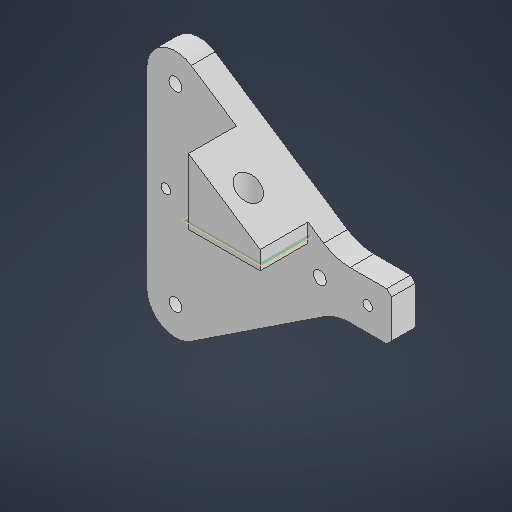
# Autodesk Inventor part: y axis something back
Saved by Autodesk Inventor 2025.1 (Build 291241000, 241)
## iProperties
Created: 2025-02-02
Part Number: y axis something back
Material: Generic
Document SubType Name: Modeling
Designer: jerem
Density: 1 g/cm^3
Appearance: Default
Author: jerem
## iProperties of the stored document y axis something back_3DPrint.ipt
Created: 2025-02-19
Part Number: y axis something back_3DPrint
Material: Generic
Document SubType Name: Modeling
Designer: jerem
Density: 1 g/cm^3
Appearance: Default
Author: jerem
Autodesk Inventor part; units mm, degrees
ref_plane "YZ Plane" through (0, 0, 0) normal (1, 0, 0) x (0, 1, 0)
ref_plane "XZ Plane" through (0, 0, 0) normal (0, 1, 0) x (-1, 0, 0)
ref_plane "XY Plane" through (0, 0, 0) normal (0, 0, 1) x (1, 0, 0)
sketch "Sketch1" plane through (0, 0, 0) normal (0, 0, 1) x (1, 0, 0)
  line L0 (0, 0) -> (30.25, 0) construction
  line L1 (0, 0) -> (-30.25, 0) construction
  line L2 (-30.25, 0) -> (-30.25, 40) construction
  line L3 (-30.25, 0) -> (-30.25, -40) construction
  circle A0 centre (-30.25, 40) radius 2.7
  circle A1 centre (-30.25, -40) radius 2.7
  circle A2 centre (30.25, 0) radius 2.7
  circle A3 centre (-30.25, 40) radius 12
  circle A4 centre (-30.25, -40) radius 12
  circle A5 centre (30.25, 0) radius 12
  line L4 (36.868172, -10.009985) -> (-23.631828, -50.009985)
  line L5 (-42.25, 40) -> (-42.25, -40)
  circle A6 centre (-34.25, 0) radius 2
  line L6 (-30.25, 0) -> (-34.25, 0) construction
  line L7 (-23.631828, 50.009985) -> (36.868172, 10.009985)
  line L8 (30.25, 0) -> (50.25, 0) construction
  circle A7 centre (50.25, 0) radius 10
  circle A8 centre (50.25, 0) radius 2
  line L9 (50.25746, 9.999997) -> (36.868172, 10.009985)
  line L10 (50.25746, -9.999997) -> (36.868172, -10.009985)
  circle A9 centre (10.25, 0) radius 2
  line L11 (50.25746, -9.999997) -> (60.257457, -9.992538)
  line L12 (60.257457, -9.992538) -> (60.242549, 9.992549)
  line L13 (60.242549, 9.992549) -> (50.25746, 9.999997)
  point P0 (-42.25, 0)
  point P1 (41.35, -4.559605)
  point P2 (41.35, 4.559605)
  point P3 (60.249997, 0.00746)
  dimension "d0" = 60.5
  dimension "d1" = 5.4
  dimension "d2" = 80
  dimension "d3" = 24
  dimension "d55" = 4
  dimension "d56" = 8
  dimension "d57" = 20
  dimension "d58" = 20
  dimension "d69" = 20
  constraints: 28 end point, 10 centre point, 10 tangent, 8 coincident, 8 point on circle, 6 equal radius, 4 horizontal, 2 collinear, 2 perpendicular, 2 vertical, 1 midpoint, 1 point on line
  measures "d0" distance of L0.end L1.end
  measures "d1" diameter of A0
  measures "d2" distance of L3.end L2.end
  measures "d3" diameter of A3
  measures "d55" diameter of A6
  measures "d56" distance of point (-42.25, 0) L6.end
  measures "d57" distance of L8.start L8.end
  measures "d58" diameter of A7
  measures "d69" distance of A9.centre L0.end
sketch "Sketch1 outline for Extrusion1" plane through (0, 0, 0) normal (0, 0, 1) x (1, 0, 0)
  arc A0 (-23.631828, 50.009985) -> (-42.25, 40) centre (-30.25, 40) ccw
  line L0 (-42.25, 40) -> (-42.25, -40)
  arc A1 (-42.25, -40) -> (-23.631828, -50.009985) centre (-30.25, -40) ccw
  line L1 (-23.631828, -50.009985) -> (36.868172, -10.009985)
  line L2 (36.868172, -10.009985) -> (60.257457, -9.992538)
  line L3 (60.257457, -9.992538) -> (60.242549, 9.992549)
  line L4 (60.242549, 9.992549) -> (36.868172, 10.009985)
  line L5 (36.868172, 10.009985) -> (-23.631828, 50.009985)
  circle A2 centre (-30.25, 40) radius 2.7
  circle A3 centre (10.25, 0) radius 2
  circle A4 centre (-34.25, 0) radius 2
  circle A5 centre (30.25, 0) radius 2.7
  circle A6 centre (-30.25, -40) radius 2.7
  circle A7 centre (50.25, 0) radius 2
extrude "Extrusion1" add sketch "Sketch1 outline for Extrusion1" against normal blind 10
fillet "Fillet1" radius 20 2 edges at (36.8682, 10.01, -5) (36.8682, -10.01, -5)
sketch "Sketch5" plane through (0, 0, 0) normal (0, 0, 1) x (1, 0, 0)
  arc A0 (-42.25, -40) -> (-23.631828, -50.009985) centre (-30.25, -40) ccw
  line L0 (-23.631828, -50.009985) -> (31.85846, -13.322191)
  arc A1 (42.873828, -10.005505) -> (31.85846, -13.322191) centre (42.888747, -30.0055) ccw
  line L1 (42.873828, -10.005505) -> (60.257457, -9.992538)
  arc A2 (31.85846, 13.322191) -> (42.873828, 10.005505) centre (42.888747, 30.0055) ccw
  line L2 (31.85846, 13.322191) -> (-23.631828, 50.009985)
  arc A3 (-23.631828, 50.009985) -> (-42.25, 40) centre (-30.25, 40) ccw
  line L3 (-42.25, 40) -> (-42.25, -40)
  circle A4 centre (-30.25, -40) radius 2.7
  circle A5 centre (30.25, 0) radius 2.7
  circle A6 centre (-34.25, 0) radius 2
  circle A7 centre (-30.25, 40) radius 2.7
  circle A8 centre (50.25, 0) radius 2
  line L4 (-4.75, 10) -> (-4.75, 37.526132)
  line L5 (-4.75, 10) -> (25.25, 10)
  line L6 (25.25, 10) -> (25.25, 17.691421)
  line L7 (60.257457, -9.992538) -> (60.242549, 9.992549)
  line L8 (60.242549, 9.992549) -> (42.873828, 10.005505)
  point P0 (10.267224, 24.242705)
  point P1 (8.658764, 37.564896)
  dimension "d64" = 10
  dimension "d65" = 5
  dimension "d66" = 30
  constraints: 6 end point, 2 point on line, 1 horizontal, 1 perpendicular, 1 vertical, 1 other
  measures "d64" distance from line of L5 A5.centre
  measures "d65" horizontal distance of L5.end A5.centre
  measures "d66" distance of L4.start L5.end
extrude "Extrusion6" add sketch "Sketch5" along normal blind 20 contours L2 L6 L5 L4
sketch "Sketch6" plane through (-4.75, 10, 0) normal (0, -1, 0) x (1, 0, 0)
  line L0 (30, 0) -> (30, 20) projected
  line L1 (0, 20) -> (30, 20) projected
  line L2 (0, 0) -> (0, 20) projected
  line L3 (13, 0) -> (17, 0) projected
  line L4 (15, 0) -> (15, 10) construction
  circle A0 centre (15, 10) radius 2
  point P0 (4.75, 0)
  dimension "d70" = 10
  dimension "d71" = 4
  constraints: 2 end point, 1 centre point, 1 coincident, 1 midpoint, 1 vertical
  measures "d70" distance of L4.start L4.end
  measures "d71" diameter of A0
ref_plane "Work Plane1" through (-4.75, 13, 0) normal (0, -1, 0) x (1, 0, 0)
extrude "Extrusion7" cut sketch "Sketch6" against normal through all
sketch "Sketch7" plane through (-4.75, 13, 0) normal (0, -1, 0) x (1, 0, 0)
  circle A0 centre (15, 10) radius 2 projected
  circle A1 centre (15, 10) radius 4.5
  point P0 (4.75, 0)
  dimension "d75" = 9
  constraints: 1 centre point, 1 coincident
  measures "d75" diameter of A1
extrude "Extrusion8" cut sketch "Sketch7" against normal through all
chamfer "Chamfer6" distance 2 angle 45 2 edges at (60.2425, 9.9925, -5) (60.2575, -9.9925, -5)
equation "\"b\" = 2"
body "Solid1"
